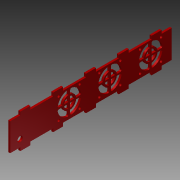
# Autodesk Inventor part: SidePanel_FanCutout2
Saved by Autodesk Inventor 2015 SP1 (Build 190203100, 203)
## iProperties
Created: 2014-08-06
Part Number: SidePanel_FanCutout2
Material: Acrylic
Document SubType Name: Modeling
Designer: Patrick Camilleri
Density: 1.188 g/cm^3
Appearance: Smooth - Red
Author: Patrick Camilleri
Autodesk Inventor part; units mm, degrees
ref_plane "YZ Plane" through (0, 0, 0) normal (1, 0, 0) x (0, 1, 0)
ref_plane "XZ Plane" through (0, 0, 0) normal (0, 1, 0) x (-1, 0, 0)
ref_plane "XY Plane" through (0, 0, 0) normal (0, 0, 1) x (1, 0, 0)
sketch "Sketch1" plane through (0, 0, 0) normal (0, 1, 0) x (-1, 0, 0)
  line L0 (21.065, 123) -> (-21.065, 123)
  line L1 (-21.065, 123) -> (-21.065, -123)
  line L2 (-21.065, -123) -> (21.065, -123)
  line L3 (21.065, -123) -> (21.065, 123)
  line L4 (21.065, 123) -> (-21.065, -123) construction
  line L5 (-21.065, 123) -> (21.065, -123) construction
  point P0 (0, 0)
  point P1 (0, 0)
  dimension "d0" = 42.13
  dimension "d1" = 246
  constraints: 12 end point, 3 midpoint, 2 parallel, 1 horizontal, 1 perpendicular
  measures "d0" distance of L2.end L1.end
  measures "d1" distance of L1.end L0.end
extrude "Extrusion1" add sketch "Sketch1" along normal blind 3
sketch "Sketch21" plane through (0, 0, 0) normal (0, -1, 0) x (1, 0, 0)
  line L0 (-21.065, 123) -> (21.065, 123) projected
  line L1 (-17, 17) -> (15, 17) construction
  line L2 (15, 17) -> (15, 49) construction
  line L3 (15, 49) -> (-17, 49) construction
  line L4 (-17, 49) -> (-17, 17) construction
  line L5 (-17, 17) -> (15, 49) construction
  line L6 (15, 17) -> (-17, 49) construction
  line L7 (0, -123.1916) -> (0, 123) construction
  line L8 (-21.065, 123) -> (21.065, 123) projected
  circle A0 centre (-1, 33) radius 18
  circle A1 centre (-1, 33) radius 10.5
  circle A2 centre (-1, 33) radius 8
  line L9 (-19, 31.75) -> (17, 31.75)
  line L10 (17, 31.75) -> (17, 34.25)
  line L11 (17, 34.25) -> (-19, 34.25)
  line L12 (-19, 34.25) -> (-19, 31.75)
  line L13 (-19, 31.75) -> (17, 34.25) construction
  line L14 (17, 31.75) -> (-19, 34.25) construction
  line L15 (-2.25, 15) -> (0.25, 15)
  line L16 (0.25, 15) -> (0.25, 51)
  line L17 (0.25, 51) -> (-2.25, 51)
  line L18 (-2.25, 51) -> (-2.25, 15)
  line L19 (-2.25, 15) -> (0.25, 51) construction
  line L20 (0.25, 15) -> (-2.25, 51) construction
  point P0 (0, 0)
  dimension "d272" = 32
  dimension "d273" = 32
  dimension "d307" = 90
  dimension "d329" = 1
  dimension "d332" = 36
  dimension "d333" = 21
  dimension "d334" = 16
  dimension "d353" = 36
  dimension "d354" = 2.5
  dimension "d355" = 2.5
  dimension "d356" = 36
  constraints: 38 end point, 9 coincident, 6 midpoint, 6 parallel, 3 centre point, 3 horizontal, 3 perpendicular, 1 point on line
  measures "d272" distance of L3.end L2.end
  measures "d273" distance of L2.end L1.end
  measures "d307" distance from line of point (-1, 33) L0
  measures "d329" distance from line of L7 point (-1, 33)
  measures "d332" diameter of A0
  measures "d333" diameter of A1
  measures "d334" diameter of A2
  measures "d353" distance of L11.end L10.end
  measures "d354" distance of L10.end L9.end
  measures "d355" distance of L17.end L16.end
  measures "d356" distance of L16.end L15.end
sketch "Sketch22" plane through (0, 0, 0) normal (0, -1, 0) x (1, 0, 0)
  line L0 (-21.065, -123) -> (-21.065, 123) projected
  line L1 (21.065, -123) -> (-21.065, -123) projected
  line L2 (21.065, 123) -> (21.065, -123) projected
  line L3 (-21.065, 123) -> (21.065, 123) projected
  line L4 (-26.065, -7.565) -> (-21.065, -7.565)
  line L5 (-21.065, -7.565) -> (-21.065, 7.565)
  line L6 (-21.065, 7.565) -> (-26.065, 7.565)
  line L7 (-26.065, 7.565) -> (-26.065, -7.565)
  line L8 (-26.065, -7.565) -> (-21.065, 7.565) construction
  line L9 (-21.065, -7.565) -> (-26.065, 7.565) construction
  line L10 (21.065, -7.565) -> (26.065, -7.565)
  line L11 (26.065, -7.565) -> (26.065, 7.565)
  line L12 (26.065, 7.565) -> (21.065, 7.565)
  line L13 (21.065, 7.565) -> (21.065, -7.565)
  line L14 (21.065, -7.565) -> (26.065, 7.565) construction
  line L15 (26.065, -7.565) -> (21.065, 7.565) construction
  point P0 (0, 0)
  point P1 (-23.565, 0)
  point P2 (-21.065, 0)
  point P3 (23.565, 0)
  point P4 (21.065, 0)
  dimension "d296" = 15.13
  dimension "d297" = 5
  dimension "d298" = 15.13
  dimension "d299" = 5
  constraints: 24 end point, 8 midpoint, 4 parallel, 2 horizontal, 2 perpendicular
  measures "d296" distance of L6.end L4.start
  measures "d297" distance of L5.end L6.end
  measures "d298" distance of L10.end L11.end
  measures "d299" distance of L11.end L12.end
extrude "Extrusion18" add sketch "Sketch22" against normal blind 3 contours L4 L7 L6 L0 | L2 L12 L11 L10
pattern_linear "Rectangular Pattern22" count 5 spacing 50 along (0, 0, 1) of "Extrusion18" first direction both ways yes
sketch "Sketch5" plane through (0, 0, 0) normal (0, -1, 0) x (1, 0, 0)
  line L0 (-21.065, 123) -> (21.065, 123) projected
  circle A0 centre (10, 108) radius 4
  line L1 (21.065, 123) -> (21.065, 107.565) projected
  point P0 (0, 0)
  dimension "d106" = 8
  dimension "d107" = 15
  dimension "d331" = 10
  constraints: 1 centre point
  measures "d106" diameter of A0
  measures "d107" distance from line of A0.centre L0
  measures "d331" horizontal distance of A0.centre point (0, 0)
extrude "Extrusion19" cut sketch "Sketch5" against normal blind 10
hole "Hole5" at (-17, 0, 49) at (15, 0, 49) at (15, 0, 17) at (-17, 0, 17) direction (0, 1, 0) diameter 4 end through all
pattern_linear "Rectangular Pattern23" count 3 spacing 62 along (0, 0, -1) of "Hole5"
extrude "Extrusion21" cut sketch "Sketch21" against normal blind 10 contours A0 L9 A1 L11 | L11 A1 L16 A0 | A0 L16 A1 L9 | L16 A1 L18 A0 | A0 L18 A1 L16 | L11 L16 A2 | A2 L9 L16 L11 | A2 L16 L9 | L18 A1 L11 A0 | L16 L11 L18 A2 | L16 L9 L18 L11 | A0 L9 A1 L18 | A2 L18 L9 L16 | L11 A1 L9 A0 | L18 L11 A2 | L18 L9 A2 L11 | A2 L9 L18
extrude "Extrusion23" add sketch "Sketch21" against normal blind 3 contours A0 L9 A1 L11 | L10 L9 A0 | A0 L11 L10 | L16 A1 L18 A0 | A0 L17 L16 | A1 L9 A2 L11 | L16 L15 A0 | A0 L18 A1 L16 | A0 L18 L17 | L16 A2 L18 A1 | A2 L9 L16 L11 | L15 L18 A0 | A1 L18 A2 L16 | L16 L11 L18 A2 | L16 L9 L18 L11 | A2 L18 L9 L16 | L11 A1 L9 A0 | A0 L12 L11 | L11 A2 L9 A1 | L18 L9 A2 L11 | L9 L12 A0
pattern_linear "Rectangular Pattern26" count 3 spacing 62 along (0, 0, -1) of "Extrusion21", "Extrusion23"
fillet "Fillet" radius 2 24 edges at (-2.25, 1.5, -46.9565) (-18.9565, 1.5, -30.25) (-18.9565, 1.5, -27.75) (16.9565, 1.5, -30.25) (16.9565, 1.5, -27.75) (0.25, 1.5, -11.0435) (-2.25, 1.5, -11.0435) (0.25, 1.5, -46.9565) (0.25, 1.5, -108.9565) (-18.9565, 1.5, -89.75) (-2.25, 1.5, -73.0435) (16.9565, 1.5, -92.25) (16.9565, 1.5, -89.75) (-2.25, 1.5, -108.9565) (0.25, 1.5, -73.0435) (-18.9565, 1.5, -92.25) (-2.25, 1.5, 15.0435) (16.9565, 1.5, 34.25) (0.25, 1.5, 50.9565) (-18.9565, 1.5, 31.75) (-18.9565, 1.5, 34.25) (0.25, 1.5, 15.0435) (-2.25, 1.5, 50.9565) (16.9565, 1.5, 31.75)
equation "\"kerf\" = 0.13"
equation "\"tab_w\" = 15"
equation "\"tab_h\" = 5"
body "Solid1"
